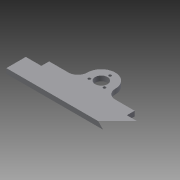
# Autodesk Inventor part: ZAxisNutMountMetal
Saved by Autodesk Inventor 2015 SP1 (Build 190203100, 203)
## iProperties
Created: 2015-01-27
Part Number: ZAxisNutMountMetal
Material: Generic
Document SubType Name: Modeling
Designer: Jack
Density: 1 g/cm^3
Appearance: Default
Vendor: Jack
Author: Jack
Title: Z Nut Mount
Autodesk Inventor part; units mm, degrees
ref_plane "YZ Plane" through (0, 0, 0) normal (1, 0, 0) x (0, 1, 0)
ref_plane "XZ Plane" through (0, 0, 0) normal (0, 1, 0) x (-1, 0, 0)
ref_plane "XY Plane" through (0, 0, 0) normal (0, 0, 1) x (1, 0, 0)
sketch "Sketch1" plane through (0, 0, 0) normal (0, 0, 1) x (1, 0, 0)
  line L0 (0, 0) -> (150, 0)
  line L1 (0, 0) -> (0, 25)
  line L2 (0, 25) -> (20, 25)
  circle A0 centre (75, 47.15) radius 8
  line L3 (20, 25) -> (20, 35)
  line L4 (20, 35) -> (61.7193, 35)
  line L5 (150, 0) -> (150, 25)
  line L6 (150, 25) -> (130, 25)
  line L7 (130, 25) -> (130, 35)
  line L8 (130, 35) -> (88.2807, 35)
  arc A1 (88.2807, 35) -> (61.7193, 35) centre (75, 47.15) ccw
  dimension "d0" = 150
  dimension "d1" = 25
  dimension "d3" = 16
  dimension "d4" = 10
  dimension "d5" = 36
  dimension "d6" = 75
  dimension "d7" = 22.15
  dimension "d19" = 20
  dimension "d20" = 20
  constraints: 18 end point, 4 perpendicular, 3 vertical, 2 centre point, 2 horizontal, 2 parallel, 2 point on circle, 1 coincident
  measures "d0" distance of L0.start L0.end
  measures "d1" distance of L0.start L1.end
  measures "d3" diameter of A0
  measures "d4" distance of L2.end L3.end
  measures "d5" diameter of A1
  measures "d6" distance from line of L5 A0.centre
  measures "d7" distance from line of A0.centre L6
  measures "d19" distance of L5.end L6.end
  measures "d20" distance of L1.end L2.end
extrude "Extrusion1" add sketch "Sketch1" along normal blind 6.35
fillet "Fillet1" radius 16 2 edges at (61.7193, 35, 3.175) (88.2807, 35, 3.175)
sketch "Sketch2" plane through (0, 0, 6.35) normal (0, 0, 1) x (1, 0, 0)
  arc A0 (92.8842, 49.1882) -> (57.1158, 49.1882) centre (75, 47.15) ccw projected
  circle A1 centre (75, 58.4) radius 1.75
  circle A2 centre (84.7428, 41.525) radius 1.75
  circle A3 centre (65.2572, 41.525) radius 1.75
  line L0 (75, 47.15) -> (75, 58.4) construction
  line L1 (75, 47.15) -> (84.7428, 41.525) construction
  line L2 (75, 47.15) -> (65.2572, 41.525) construction
  dimension "d11" = 120
  dimension "d12" = 120
  dimension "d13" = 11.25
  dimension "d14" = 11.25
  dimension "d15" = 11.25
  dimension "d16" = 3.5
  constraints: 6 end point, 3 centre point, 3 coincident, 2 equal radius, 1 vertical
  measures "d11" angle of L0 L1
  measures "d12" angle of L1 L2
  measures "d13" distance of L0.start L2.end
  measures "d14" distance of L0.start L1.end
  measures "d15" distance of L0.start L0.end
  measures "d16" diameter of A1
extrude "Extrusion2" cut sketch "Sketch2" against normal up to next
body "Solid1"
